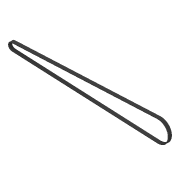
# Autodesk Inventor part: Tandriem20naar60T-696mm
Saved by Autodesk Inventor 2020.3 (Build 243373000, 373)
## iProperties
Created: 2020-05-20
Part Number: Tandriem20naar60T-696mm
Material: Rubber
Document SubType Name: Modeling
Designer: Svend
Density: 0.93 g/cm^3
Appearance: Rubber - Black
Author: Svend
Autodesk Inventor part; units mm, degrees
ref_plane "YZ Plane" through (0, 0, 0) normal (1, 0, 0) x (0, 1, 0)
ref_plane "XZ Plane" through (0, 0, 0) normal (0, 1, 0) x (-1, 0, 0)
ref_plane "XY Plane" through (0, 0, 0) normal (0, 0, 1) x (1, 0, 0)
sketch "Sketch1" plane through (0, 0, 0) normal (0, 0, 1) x (1, 0, 0)
  arc A0 (-0.2852, 5.9932) -> (-0.2852, -5.9932) centre (0, 0) ccw
  arc A1 (269.4505, -18.8287) -> (269.4505, 18.8287) centre (270.3465, 0) ccw
  line L0 (269.4505, 18.8287) -> (-0.2852, 5.9932)
  line L1 (-0.2852, -5.9932) -> (269.4505, -18.8287)
  line L2 (-0.347, 7.2917) -> (269.3887, 20.1272)
  arc A2 (269.3887, -20.1272) -> (269.3887, 20.1272) centre (270.3465, 0) ccw
  line L3 (269.3887, -20.1272) -> (-0.347, -7.2917)
  arc A3 (-0.347, 7.2917) -> (-0.347, -7.2917) centre (0, 0) ccw
  dimension "d0" = 12
  dimension "d1" = 37.7
  dimension "d3" = 1.3
  dimension "d9" = 270.3465
  constraints: 8 end point, 8 point on circle, 4 centre point, 4 tangent, 1 coincident, 1 horizontal alignment, 3 other
  measures "d0" diameter of A0
  measures "d1" diameter of A1
  measures "d3" distance between parallel lines of L0 L2
  measures "d9" distance of A0.centre A1.centre
extrude "Extrusion1" add sketch "Sketch1" along normal mid plane 6
chamfer "Chamfer1" distance 0.2 angle 45 16 edges at (289.1965, 0, 3) (134.5826, -12.411, 3) (-6, 0, 3) (134.5826, 12.411, 3) (289.1965, 0, -3) (134.5826, 12.411, -3) (-6, 0, -3) (134.5826, -12.411, -3) (290.4965, 0, 3) (134.5209, 13.7095, 3) (-7.3, 0, 3) (134.5209, -13.7095, 3) (290.4965, 0, -3) (134.5209, -13.7095, -3) (-7.3, 0, -3) (134.5209, 13.7095, -3)
body "Solid1"
